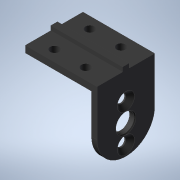
# Autodesk Inventor part: 03_MotorHolder
Saved by Autodesk Inventor 2021 (Build 250183000, 183)
## iProperties
Created: 2021-03-22
Part Number: 03_MotorHolder
Material: Generisch
Document SubType Name: Modeling
Designer: User
Density: 1 g/cm^3
Appearance: Vorgabe
Author: User
## iProperties of the stored document _3D-Druck.ipt
Created: 2021-08-11
Part Number: _3D-Druck
Material: Generisch
Document SubType Name: Modeling
Designer: User
Density: 1 g/cm^3
Appearance: Vorgabe
Author: User
Autodesk Inventor part; units mm, degrees
ref_plane "YZ Plane" through (0, 0, 0) normal (1, 0, 0) x (0, 1, 0)
ref_plane "XZ Plane" through (0, 0, 0) normal (0, 1, 0) x (-1, 0, 0)
ref_plane "XY Plane" through (0, 0, 0) normal (0, 0, 1) x (1, 0, 0)
derived "00_Mastersketch.ipt"
sketch "01_caseBottom" plane through (0, 0, 0) normal (0, 1, 0) x (-1, 0, 0)
  circle A0 centre (0, 0) radius 110
  line L0 (-11, 12.5) -> (-64, 12.5) construction
  line L1 (-64, 12.5) -> (-64, -12.5) construction
  line L2 (-64, -12.5) -> (-11, -12.5) construction
  line L3 (-11, -12.5) -> (-11, 12.5) construction
  line L4 (177.1148, 0) -> (-157.8525, 0)
  line L5 (0, -205.8736) -> (0, 465.2416)
  line L6 (-64, -13.15) -> (-67, -13.15) construction
  line L7 (-67, -13.15) -> (-67, 13.15) construction
  line L8 (-67, 13.15) -> (-64, 13.15) construction
  line L9 (-64, 13.15) -> (-64, -13.15) construction
  line L10 (-67, -2) -> (-76, -2) construction
  line L11 (-76, -2) -> (-76, 2) construction
  line L12 (-76, 2) -> (-67, 2) construction
  line L13 (-67, 2) -> (-67, 3.5) construction
  line L14 (-67, 3.5) -> (-64, 3.5) construction
  line L15 (-67, -2) -> (-67, -3.5) construction
  line L16 (-67, -3.5) -> (-64, -3.5) construction
  line L17 (-67, -5.5) -> (-79, -5.5) construction
  line L18 (-79, -5.5) -> (-79, 5.5) construction
  line L19 (-79, 5.5) -> (-67, 5.5) construction
  line L20 (-67, 5.5) -> (-67, -5.5) construction
  line L21 (-79, 5.5) -> (-79, 6) construction
  line L22 (-79, 6) -> (-85, 6) construction
  line L23 (-85, 6) -> (-85, -6) construction
  line L24 (-85, -6) -> (-79, -6) construction
  line L25 (-79, -6) -> (-79, -5.5) construction
  line L26 (-71, 33.5) -> (-71, -33.5) construction
  line L27 (-71, -33.5) -> (-97, -33.5) construction
  line L28 (-97, -33.5) -> (-97, 33.5) construction
  line L29 (-97, 33.5) -> (-71, 33.5) construction
  line L30 (-97, -33.5) -> (-85, -16) construction
  line L31 (-85, -16) -> (-85, 16) construction
  line L32 (-85, 16) -> (-97, 33.5) construction
  line L33 (-11, 6) -> (-4, 6) construction
  line L34 (-4, 6) -> (-4, -6) construction
  line L35 (-4, -6) -> (-11, -6) construction
  line L36 (40.2623, 315.7467) -> (40.2623, 365.7467) construction
  line L37 (43.2623, 368.7467) -> (122.2623, 368.7467) construction
  line L38 (125.2623, 365.7467) -> (125.2623, 366.8467) construction
  line L39 (125.2623, 366.8467) -> (129.2623, 366.8467) construction
  line L40 (129.2623, 366.8467) -> (129.2623, 350.9467) construction
  line L41 (129.2623, 350.9467) -> (125.2623, 350.9467) construction
  line L42 (125.2623, 350.9467) -> (125.2623, 347.3967) construction
  line L43 (125.2623, 347.3967) -> (129.2623, 347.3967) construction
  line L44 (129.2623, 347.3967) -> (129.2623, 332.4967) construction
  line L45 (129.2623, 332.4967) -> (125.2623, 332.4967) construction
  line L46 (125.2623, 332.4967) -> (125.2623, 329.1967) construction
  line L47 (125.2623, 329.1967) -> (129.2623, 329.1967) construction
  line L48 (129.2623, 329.1967) -> (129.2623, 314.2967) construction
  line L49 (129.2623, 314.2967) -> (125.2623, 314.2967) construction
  line L50 (125.2623, 314.2967) -> (125.2623, 315.7467) construction
  line L51 (122.2623, 312.7467) -> (97.5873, 312.7467) construction
  line L52 (97.5873, 312.7467) -> (97.5873, 308.9047) construction
  line L53 (97.5873, 308.9047) -> (91.5873, 308.9047) construction
  line L54 (91.5873, 308.9047) -> (91.5873, 312.7467) construction
  line L55 (91.5873, 312.7467) -> (83.3243, 312.7467) construction
  line L56 (83.3243, 312.7467) -> (83.3243, 309.2487) construction
  line L57 (83.3243, 309.2487) -> (76.8243, 309.2487) construction
  line L58 (76.8243, 309.2487) -> (76.8243, 312.7467) construction
  line L59 (76.8243, 312.7467) -> (69.8243, 312.7467) construction
  line L60 (69.8243, 312.7467) -> (69.8243, 309.2487) construction
  line L61 (69.8243, 309.2487) -> (63.3243, 309.2487) construction
  line L62 (63.3243, 309.2487) -> (63.3243, 312.7467) construction
  line L63 (63.3243, 312.7467) -> (56.1843, 312.7467) construction
  line L64 (56.1843, 312.7467) -> (56.1843, 309.2487) construction
  line L65 (56.1843, 309.2487) -> (47.2443, 309.2487) construction
  line L66 (47.2443, 309.2487) -> (47.2443, 312.7467) construction
  line L67 (47.2443, 312.7467) -> (43.2623, 312.7467) construction
  arc A1 (43.2623, 368.7467) -> (40.2623, 365.7467) centre (43.2623, 365.7467) ccw construction
  arc A2 (125.2623, 365.7467) -> (122.2623, 368.7467) centre (122.2623, 365.7467) ccw construction
  arc A3 (122.2623, 312.7467) -> (125.2623, 315.7467) centre (122.2623, 315.7467) ccw construction
  arc A4 (40.2623, 315.7467) -> (43.2623, 312.7467) centre (43.2623, 315.7467) ccw construction
  circle A5 centre (43.7623, 365.2467) radius 1.35 construction
  circle A6 centre (101.7623, 365.2467) radius 1.35 construction
  circle A7 centre (101.7623, 316.2467) radius 1.35 construction
  circle A8 centre (43.7623, 316.2467) radius 1.35 construction
  circle A9 centre (43.7623, 365.2467) radius 3 construction
  circle A10 centre (43.7623, 316.2467) radius 3 construction
  circle A11 centre (101.7623, 365.2467) radius 3 construction
  circle A12 centre (101.7623, 316.2467) radius 3 construction
  line L68 (43.7623, 316.2467) -> (43.7623, 365.2467) construction
  line L69 (43.7623, 365.2467) -> (101.7623, 365.2467) construction
  line L70 (101.7623, 365.2467) -> (101.7623, 316.2467) construction
  line L71 (101.7623, 316.2467) -> (43.7623, 316.2467) construction
  circle A13 centre (0, 0) radius 107.6
  line L72 (-85, -6.25) -> (-71, -6.25) construction
  line L73 (-85, 6.25) -> (-71, 6.25) construction
  line L74 (19, -102) -> (-19, -102)
  line L75 (-19, -102) -> (-19, -69)
  line L76 (-19, -69) -> (19, -69)
  line L77 (19, -69) -> (19, -102)
  line L78 (-99.3342, 35.8342) -> (-99.3342, -35.8342)
  line L79 (-99.3342, -35.8342) -> (-68.6658, -35.8342)
  line L80 (-68.6658, -35.8342) -> (-68.6658, 35.8342)
  line L81 (-68.6658, 35.8342) -> (-99.3342, 35.8342)
  line L82 (-64, 13.15) -> (-34.3, 13.15) construction
  line L83 (-34.3, 13.15) -> (-34.3, -13.15) construction
  line L84 (-34.3, -13.15) -> (-64, -13.15) construction
  circle A14 centre (-49.7, 0) radius 5 construction
  circle A15 centre (-42.6, -8.05) radius 1.8 construction
  circle A16 centre (-56.8, -8.05) radius 1.8 construction
  circle A17 centre (-56.8, 8.05) radius 1.8 construction
  circle A18 centre (-42.6, 8.05) radius 1.8 construction
  line L85 (-42.6, -8.05) -> (-42.6, 8.05) construction
  line L86 (-42.6, 8.05) -> (-56.8, 8.05) construction
  line L87 (-56.8, 8.05) -> (-56.8, -8.05) construction
  line L88 (-56.8, -8.05) -> (-42.6, -8.05) construction
  line L89 (-42.6, 8.05) -> (-56.8, -8.05) construction
  line L90 (-56.8, 8.05) -> (-42.6, -8.05) construction
  line L91 (-64, 8.6) -> (-67, 8.6) construction
  line L92 (-64, -8.6) -> (-67, -8.6) construction
  circle A19 centre (-42.6, -8.05) radius 2.1
  circle A20 centre (-42.6, 8.05) radius 2.1
  circle A21 centre (-56.8, 8.05) radius 2.1
  circle A22 centre (-56.8, -8.05) radius 2.1
  circle A23 centre (-49.7, 0) radius 5
  line L93 (-34.3, 0) -> (-67, 0) construction
  line L94 (-68.6658, -13.55) -> (-63.9618, -13.55)
  line L95 (-63.9618, -13.55) -> (-63.9618, 13.55)
  line L96 (-63.9618, 13.55) -> (-68.6658, 13.55)
  line L97 (0, 0) -> (0, 110) construction
  circle A24 centre (0, 105) radius 5
  line L98 (-99.3342, -35.8342) -> (-101.2155, -36.5128) construction
  line L99 (0, -69) -> (0, -102) construction
  circle A25 centre (15, -97.5) radius 2.15 construction
  circle A26 centre (15, -73.5) radius 2.15 construction
  circle A27 centre (-15, -73.5) radius 2.15 construction
  circle A28 centre (-15, -97.5) radius 2.15 construction
  line L100 (15, -73.5) -> (15, -97.5) construction
  line L101 (15, -97.5) -> (-15, -97.5) construction
  line L102 (-15, -97.5) -> (-15, -73.5) construction
  line L103 (-15, -73.5) -> (15, -73.5) construction
  line L104 (19, -85.5) -> (-19, -85.5) construction
  point P0 (-64, 0)
  point P1 (-76, 0)
  point P2 (-11, 0)
  point P3 (-79, 0)
  point P4 (-85, 0)
  point P5 (-85, 0)
  point P6 (-71, 0)
  point P7 (-4, 0)
  point P8 (40.2623, 312.7467)
  point P9 (125.2623, 312.7467)
  dimension "d50" = 0.3
  measures "d50" radial gap between concentric circles of A15 A19
sketch "06_motorHolderSketch" plane through (49.7, 0, 0) normal (0, 0, 1) x (1, 0, 0)
  line L0 (14.3, 0) -> (-15.4, 0) construction
  line L1 (17.3, 0) -> (14.3, 0) construction
  line L2 (17.3, -31.1) -> (17.3, 3) construction
  line L3 (17.3, 3) -> (-15.4, 3) construction
  line L4 (-15.4, 3) -> (-15.4, 0) construction
  line L5 (-15.4, 0) -> (14.8, 0) construction
  line L6 (14.8, 0) -> (14.8, -31.1) construction
  line L7 (14.8, -31.1) -> (17.3, -31.1) construction
  line L8 (14.8, -17.95) -> (17.3, -17.95) construction
  line L9 (14.8, -31.1) -> (17.3, -31.1)
  line L10 (17.3, -31.1) -> (17.3, 3)
  line L11 (17.3, 3) -> (-15.4, 3)
  line L12 (-15.4, 3) -> (-15.4, 0)
  line L13 (-15.4, 0) -> (14.8, 0)
  line L14 (14.8, 0) -> (14.8, -31.1)
  point P0 (-49.7, 0)
extrude "Extrusion2" add sketch "06_motorHolderSketch" along normal mid plane 26.3
extrude "Extrusion3" cut sketch "01_caseBottom" along normal through all contours A19 | A20 | A21 | A22
sketch "Skizze6" plane through (67, -31.1, 13.15) normal (1, 0, 0) x (0, 0, -1)
  circle A0 centre (13.15, 13.15) radius 4.2
  circle A1 centre (4.55, 13.15) radius 1.95
  circle A2 centre (21.75, 13.15) radius 1.95
  line L0 (4.55, 13.15) -> (21.75, 13.15) construction
  line L1 (4.55, 13.15) -> (4.55, 31.1) construction
  line L2 (21.75, 13.15) -> (21.75, 31.1) construction
  line L3 (13.15, 21.75) -> (13.15, 4.55) construction
  circle A3 centre (13.15, 21.75) radius 1.95
  circle A4 centre (13.15, 4.55) radius 1.95
  point P0 (13.15, 31.1)
  point P1 (4.55, 31.1)
  dimension "d40" = 8.4
  dimension "d41" = 3.9
  constraints: 8 end point, 5 centre point, 5 coincident, 3 equal radius, 3 vertical, 2 midpoint, 1 horizontal, 1 perpendicular, 1 other
  measures "d40" diameter of A0
  measures "d41" diameter of A2
extrude "Extrusion4" cut sketch "Skizze6" against normal through all contours A0 | A3 | A4
full round fillet "Rundung2" first side at (55.2667, 2, 13.15) centre faces at (65.3333, -31.1, -4.3833) second side at (55.2667, 2, -13.15)
chamfer "Fase2" distance 2 angle 45 2 edges at (67, -9.35, 1.95) (67, -26.55, 1.95)
chamfer "Fase3" distance 0.4 angle 45 1 edges at (67, -17.95, 4.2)
sketch "Skizze7" plane through (0, 0, 0) normal (0, 0, 1) x (1, 0, 0)
  line L0 (64.5, 0) -> (64.5, -17.95) projected
  line L1 (34.3, 0) -> (64.5, 0) projected
  line L2 (67, 3) -> (34.3, 3) projected
  line L3 (67, -17.95) -> (67, 3) projected
  line L4 (67, -17.95) -> (67, -31.1) projected
  line L5 (64.5, -31.1) -> (64.5, -17.95) projected
  line L6 (34.3, 3) -> (34.3, 0) projected
  line L7 (34.3, 3) -> (34.3, 5)
  line L8 (34.3, 5) -> (67, 5)
  line L9 (67, 5) -> (67, 3)
  point P0 (0, 0)
  dimension "d51" = 2
  constraints: 6 end point, 2 collinear, 1 perpendicular, 1 point on line
  measures "d51" distance between parallel lines of L8 L2
extrude "Extrusion5" add sketch "Skizze7" along normal mid plane 3
equation "\"d36\" = motorHolderH"
equation "\"motorHolderH\" = 26.3"
